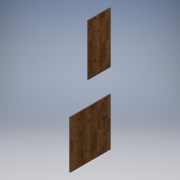
# Autodesk Inventor part: pared_lateral
Saved by Autodesk Inventor 2016 (Build 200138000, 138)
## iProperties
Created: 2015-11-25
Part Number: pared_lateral
Material: Generic
Document SubType Name: Modeling
Designer: Daniela
Density: 1 g/cm^3
Appearance: Glossy - Black
Author: Daniela
Autodesk Inventor part; units mm, degrees
ref_plane "YZ Plane" through (0, 0, 0) normal (1, 0, 0) x (0, 1, 0)
ref_plane "XZ Plane" through (0, 0, 0) normal (0, 1, 0) x (-1, 0, 0)
ref_plane "XY Plane" through (0, 0, 0) normal (0, 0, 1) x (1, 0, 0)
sketch "Sketch1" plane through (0, 0, 0) normal (1, 0, 0) x (0, 1, 0)
  line L0 (0, 0) -> (0, 80) construction
  line L1 (0, 80) -> (-10, 80) construction
  line L2 (-10, 80) -> (-690, 80)
  line L3 (-690, 80) -> (-690, 890)
  line L4 (-690, 890) -> (-10, 890)
  line L5 (-10, 890) -> (-10, 80)
  line L6 (-10, 890) -> (-10, 1290) construction
  line L7 (-10, 1290) -> (-390, 1290)
  line L8 (-390, 1290) -> (-390, 2010)
  line L9 (-390, 2010) -> (-10, 2010)
  line L10 (-10, 2010) -> (-10, 1290)
  dimension "d0" = 80
  dimension "espesor" = 10
  dimension "ancho" = 680
  dimension "h_inf" = 810
  dimension "h_esp" = 400
  dimension "profundidad" = 380
  dimension "alto_sup" = 720
  constraints: 22 end point, 4 parallel, 3 perpendicular, 2 horizontal, 2 vertical
  measures "d0" distance of L0.start L0.end
  measures "espesor" distance of L0.end L1.end
  measures "ancho" distance of L3.end L4.end
  measures "h_inf" distance of L2.end L3.end
  measures "h_esp" distance of L4.end L6.end
  measures "profundidad" distance of L8.end L9.end
  measures "alto_sup" distance of L7.end L8.end
extrude "Extrusion1" add sketch "Sketch1" against normal blind 10
equation "\"d7\" = espesor"
body "Solid1"
